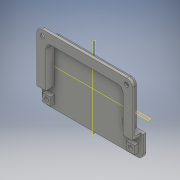
# Autodesk Inventor part: case_back
Saved by Autodesk Inventor 2016 (Build 200138000, 138)
## iProperties
Created: 2018-08-02
Part Number: case_back
Material: Generic
Document SubType Name: Modeling
Designer: Luke
Density: 1 g/cm^3
Appearance: Default
Author: Luke
Autodesk Inventor part; units mm, degrees
ref_plane "YZ Plane" through (0, 0, 0) normal (1, 0, 0) x (0, 1, 0)
ref_plane "XZ Plane" through (0, 0, 0) normal (0, 1, 0) x (-1, 0, 0)
ref_plane "XY Plane" through (0, 0, 0) normal (0, 0, 1) x (1, 0, 0)
sketch "Sketch1" plane through (0, 0, 0) normal (0, 1, 0) x (-1, 0, 0)
  line L0 (0, 0) -> (-74.5, 0)
  line L1 (-74.5, 0) -> (-74.5, 54.5)
  line L2 (-74.5, 54.5) -> (0, 54.5)
  line L3 (0, 54.5) -> (0, 0)
  dimension "d0" = 74.5
  dimension "d1" = 54.5
  constraints: 8 end point, 2 parallel, 1 horizontal, 1 perpendicular
  measures "d0" distance of L0.start L0.end
  measures "d1" distance of L0.end L1.end
extrude "Extrusion1" add sketch "Sketch1" along normal blind 2
ref_plane "Work Plane1" through (0, 0, 27.25) normal (0, 0, 1) x (1, 0, 0)
ref_plane "Work Plane2" through (37.25, 0, 0) normal (-1, 0, 0) x (0, 0, 1)
sketch "Sketch2" plane through (0, 2, 0) normal (0, 1, 0) x (1, 0, 0)
  line L0 (37.25, -65.4) -> (37.25, 10.9) construction
  line L1 (89.4, -27.25) -> (-14.9, -27.25) construction
  line L2 (6.25, -6.25) -> (68.25, -6.25) construction
  line L3 (68.25, -6.25) -> (68.25, -48.25) construction
  line L4 (68.25, -48.25) -> (6.25, -48.25) construction
  line L5 (6.25, -48.25) -> (6.25, -6.25) construction
  circle A0 centre (6.25, -6.25) radius 1.5
  circle A1 centre (68.25, -6.25) radius 1.5
  point P0 (0, 0)
  dimension "d4" = 62
  dimension "d5" = 42
  dimension "d6" = 3
  dimension "d7" = 3
  constraints: 8 end point, 2 centre point, 2 coincident, 2 parallel, 1 horizontal, 1 perpendicular, 2 other
  measures "d4" distance of L2.start L2.end
  measures "d5" distance of L2.end L3.end
  measures "d6" diameter of A0
  measures "d7" diameter of A1
sketch "Sketch3" plane through (0, 2, 0) normal (0, 1, 0) x (1, 0, 0)
  line L0 (74.5, 0) -> (0, 0) projected
  line L1 (0, 0) -> (0, -54.5) projected
  line L2 (0, -54.5) -> (74.5, -54.5) projected
  line L3 (74.5, -54.5) -> (74.5, 0) projected
  line L4 (0, -54.5) -> (0, 0) projected
  line L5 (0, -16.5) -> (6.75, -16.5)
  line L6 (6.75, -16.5) -> (6.75, -47.5)
  line L7 (6.75, -47.5) -> (67.75, -47.5)
  line L8 (67.75, -47.5) -> (67.75, -16.5)
  line L9 (67.75, -16.5) -> (74.5, -16.5)
  line L10 (37.25, -65.4) -> (37.25, 10.9) construction
  dimension "d12" = 61
  dimension "d13" = 7
  dimension "d14" = 38
  constraints: 10 end point, 4 perpendicular, 4 point on line, 1 other
  measures "d12" distance of L6.end L7.end
  measures "d13" distance between parallel lines of L2 L7
  measures "d14" distance between parallel lines of L2 L5
extrude "Extrusion3" cut sketch "Sketch3" against normal up to surface (2 mm away) contours L3 L2 L1 L5 L6 L7 L8 L9
extrude "Extrusion4" cut sketch "Sketch2" against normal up to surface (2 mm away)
sketch "Sketch4" plane through (0, 0, 0) normal (0, -1, 0) x (1, 0, 0)
  line L0 (6.75, 16.5) -> (0, 16.5) projected
  line L1 (6.75, 47.5) -> (6.75, 16.5) projected
  line L2 (67.75, 47.5) -> (6.75, 47.5) projected
  line L3 (67.75, 16.5) -> (67.75, 47.5) projected
  line L4 (74.5, 16.5) -> (67.75, 16.5) projected
  line L5 (0, 16.5) -> (0, 0) projected
  line L6 (74.5, 0) -> (74.5, 16.5) projected
  line L7 (8.75, 14.5) -> (8.75, 45.5)
  line L8 (8.75, 45.5) -> (65.75, 45.5)
  line L9 (65.75, 45.5) -> (65.75, 14.5)
  line L10 (65.75, 14.5) -> (72.5, 14.5)
  line L11 (72.5, 14.5) -> (72.5, 16.5)
  line L12 (67.75, 16.5) -> (74.5, 16.5) projected
  line L13 (8.75, 14.5) -> (2, 14.5)
  line L14 (2, 14.5) -> (2, 16.5)
  dimension "d20" = 2
  dimension "d21" = 2
  dimension "d22" = 2
  dimension "d25" = 2
  dimension "d26" = 2
  dimension "d27" = 2
  constraints: 14 end point, 4 perpendicular, 2 horizontal, 2 point on line, 1 collinear
  measures "d20" distance between parallel lines of L3 L9
  measures "d21" distance between parallel lines of L2 L8
  measures "d22" distance between parallel lines of L1 L7
  measures "d25" distance between parallel lines of L5 L14
  measures "d26" distance between parallel lines of L6 L11
  measures "d27" distance between parallel lines of L4 L10
extrude "Extrusion5" add sketch "Sketch4" along normal blind 4
sketch "Sketch5" plane through (67.75, 2, 47.5) normal (1, 0, 0) x (0, 0, -1)
  line L0 (31, 0) -> (31, -6) construction
  line L1 (0, 0) -> (31, 0) construction
  line L2 (0, 0) -> (0, -6) construction
  line L3 (31, -6) -> (0, -6) construction
  circle A0 centre (27, -2.75) radius 1.25
  point P0 (47.5, -2)
  dimension "d28" = 2.5
  dimension "d29" = 2.75
  dimension "d30" = 4
  constraints: 1 centre point
  measures "d28" diameter of A0
  measures "d29" distance from line of L1 A0.centre
  measures "d30" distance from line of L0 A0.centre
extrude "Extrusion6" cut sketch "Sketch5" against normal up to surface (2 mm away)
sketch "Sketch6" plane through (65.75, -4, 14.5) normal (-1, 0, 0) x (0, 0, 1)
  arc A0 (5, 4) -> (7, 4) centre (6, 3.25) ccw projected
  line L0 (0, 4) -> (5, 4) projected
  line L1 (7, 4) -> (31, 4) projected
  line L2 (8, 4) -> (4, 4)
  line L3 (4, 4) -> (4, 1)
  line L4 (4, 1) -> (8, 1)
  line L5 (8, 1) -> (8, 4)
  line L6 (6, 3.25) -> (6, 4) construction
  point P0 (-14.5, 4)
  dimension "d33" = 4
  dimension "d34" = 3
  constraints: 10 end point, 2 parallel, 2 perpendicular, 1 horizontal, 1 midpoint, 1 point on line, 1 other
  measures "d33" distance of L3.end L4.end
  measures "d34" distance of L2.end L3.end
extrude "Extrusion7" add sketch "Sketch6" along normal blind 3.5
sketch "Sketch7" plane through (65.75, -0.75, 20.5) normal (1, 0, 0) x (0, 0, -1)
  circle A0 centre (0, 0) radius 1.25 projected
  point P0 (20.5, 0.75)
extrude "Extrusion8" cut sketch "Sketch7" against normal blind 3
sketch "Sketch8" plane through (0, -4, 0) normal (0, -1, 0) x (1, 0, 0)
  line L0 (6.75, 16.5) -> (2, 16.5) projected
  line L1 (2, 16.5) -> (2, 14.5) projected
  line L2 (2, 14.5) -> (8.75, 14.5) projected
  line L3 (8.75, 14.5) -> (8.75, 45.5) projected
  line L4 (8.75, 45.5) -> (65.75, 45.5) projected
  line L5 (65.75, 45.5) -> (65.75, 14.5) projected
  line L6 (65.75, 14.5) -> (72.5, 14.5) projected
  line L7 (72.5, 14.5) -> (72.5, 16.5) projected
  line L8 (72.5, 16.5) -> (67.75, 16.5) projected
  line L9 (67.75, 16.5) -> (67.75, 47.5) projected
  line L10 (67.75, 47.5) -> (6.75, 47.5) projected
  line L11 (6.75, 47.5) -> (6.75, 16.5) projected
  line L12 (72.5, 16.5) -> (72.5, 52.5)
  line L13 (72.5, 52.5) -> (2, 52.5)
  line L14 (2, 52.5) -> (2, 16.5)
  point P0 (0, 0)
  dimension "d39" = 52.5
  constraints: 6 end point, 2 perpendicular, 1 vertical
  measures "d39" distance from line of L13 point (0, 0)
extrude "Extrusion9" add sketch "Sketch8" along normal blind 2
fillet "Fillet1" radius 4 4 edges at (0, 1, 0) (74.5, 1, 0) (2, -5, 52.5) (72.5, -5, 52.5)
fillet "Fillet2" radius 4 4 edges at (6.75, -1, 47.5) (67.75, -1, 47.5) (8.75, -3, 45.5) (65.75, -3, 45.5)
sketch "Sketch9" plane through (0, 0, 0) normal (0, -1, 0) x (1, 0, 0)
  circle A0 centre (68.25, 6.25) radius 1.5 projected
  circle A1 centre (6.25, 6.25) radius 1.5 projected
  line L0 (71.25, 9.25) -> (65.25, 9.25)
  line L1 (65.25, 9.25) -> (65.25, 3.25)
  line L2 (65.25, 3.25) -> (71.25, 3.25)
  line L3 (71.25, 3.25) -> (71.25, 9.25)
  line L4 (71.25, 9.25) -> (65.25, 3.25) construction
  line L5 (65.25, 9.25) -> (71.25, 3.25) construction
  line L6 (9.25, 9.25) -> (3.25, 9.25)
  line L7 (3.25, 9.25) -> (3.25, 3.25)
  line L8 (3.25, 3.25) -> (9.25, 3.25)
  line L9 (9.25, 3.25) -> (9.25, 9.25)
  line L10 (9.25, 9.25) -> (3.25, 3.25) construction
  line L11 (3.25, 9.25) -> (9.25, 3.25) construction
  point P0 (0, 0)
  dimension "d44" = 6
  dimension "d45" = 6
  dimension "d46" = 6
  dimension "d47" = 6
  constraints: 24 end point, 4 midpoint, 4 parallel, 2 horizontal, 2 perpendicular
  measures "d44" distance of L1.end L2.end
  measures "d45" distance of L0.end L1.end
  measures "d46" distance of L8.end L6.start
  measures "d47" distance of L7.end L8.end
extrude "Extrusion10" add sketch "Sketch9" along normal blind 3
sketch "Sketch10" plane through (0, 2, 0) normal (0, 1, 0) x (1, 0, 0)
  circle A0 centre (68.25, -6.25) radius 1.5 projected
  circle A1 centre (6.25, -6.25) radius 1.5 projected
  point P0 (0, 0)
extrude "Extrusion11" add sketch "Sketch10" against normal blind 1
sketch "Sketch11" plane through (0, -4, 0) normal (0, 1, 0) x (1, 0, 0)
  circle A0 centre (6.25, -6.25) radius 1.5 construction
  circle A1 centre (68.25, -6.25) radius 1.5 construction
  circle A2 centre (68.25, -6.25) radius 1.5 construction
  line L0 (6.25, -6.25) -> (68.25, -6.25) construction
  line L1 (68.25, -6.25) -> (68.25, -48.25) construction
  line L2 (68.25, -48.25) -> (6.25, -48.25) construction
  line L3 (6.25, -48.25) -> (6.25, -6.25) construction
  circle A3 centre (6.25, -48.25) radius 1.6
  circle A4 centre (68.25, -48.25) radius 1.6
  point P0 (0, 0)
  dimension "d52" = 3.2
  dimension "d53" = 3.2
  dimension "d54" = 42
  constraints: 8 end point, 3 coincident, 2 centre point, 2 parallel, 1 horizontal, 1 perpendicular
  measures "d52" diameter of A3
  measures "d53" diameter of A4
  measures "d54" distance of L0.end L1.end
extrude "Extrusion12" cut sketch "Sketch11" against normal up to surface (2 mm away)
sketch "Sketch12" plane through (0, -4, 0) normal (0, 1, 0) x (1, 0, 0)
  circle A0 centre (6.25, -48.25) radius 1.6 projected
  circle A1 centre (68.25, -48.25) radius 1.6 projected
  line L0 (4.5179, -45.25) -> (7.9821, -45.25)
  line L1 (7.9821, -45.25) -> (9.7141, -48.25)
  line L2 (9.7141, -48.25) -> (7.9821, -51.25)
  line L3 (7.9821, -51.25) -> (4.5179, -51.25)
  line L4 (4.5179, -51.25) -> (2.7859, -48.25)
  line L5 (2.7859, -48.25) -> (4.5179, -45.25)
  line L6 (69.9821, -45.25) -> (71.7141, -48.25)
  line L7 (71.7141, -48.25) -> (69.9821, -51.25)
  line L8 (69.9821, -51.25) -> (66.5179, -51.25)
  line L9 (66.5179, -51.25) -> (64.7859, -48.25)
  line L10 (64.7859, -48.25) -> (66.5179, -45.25)
  line L11 (66.5179, -45.25) -> (69.9821, -45.25)
  line L12 (68.5, -52.5) -> (6, -52.5) construction
  point P0 (0, 0)
  dimension "d57" = 6
  dimension "d58" = 6
  constraints: 24 end point, 2 coincident, 1 parallel, 1 point on line, 26 other
  measures "d57" distance between parallel lines of L3 L0
  measures "d58" distance between parallel lines of L8 L11
extrude "Extrusion13" cut sketch "Sketch12" along normal blind 3 and the other way blind 1
equation "\"d7\" = d6"
equation "\"d21\" = d20"
equation "\"d22\" = d21"
equation "\"d26\" = d25"
equation "\"d45\" = d44"
equation "\"d46\" = d45"
equation "\"d47\" = d45"
equation "\"d58\" = d57"
body "Solid1"
